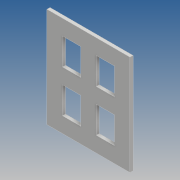
# Autodesk Inventor part: bandeja componentes
Saved by Autodesk Inventor 2017 (Build 210142000, 142)
## iProperties
Part Number: bandeja componentes
Material: Genérico
Document SubType Name: Modeling
Designer: FABLAB
Density: 1 g/cm^3
Appearance: Valor por defecto
Description: Aluminio compuesto routeado CNC
Author: FABLAB
Autodesk Inventor part; units mm, degrees
ref_plane "YZ Plane" through (0, 0, 0) normal (1, 0, 0) x (0, 1, 0)
ref_plane "XZ Plane" through (0, 0, 0) normal (0, 1, 0) x (-1, 0, 0)
ref_plane "XY Plane" through (0, 0, 0) normal (0, 0, 1) x (1, 0, 0)
sketch "Boceto1" plane through (0, 0, 0) normal (0, 1, 0) x (-1, 0, 0)
  line L0 (54, 65) -> (-54, 65)
  line L1 (-54, 65) -> (-54, -65)
  line L2 (-54, -65) -> (54, -65)
  line L3 (54, -65) -> (54, 65)
  line L4 (34, 45) -> (10, 45)
  line L5 (10, 45) -> (10, 10)
  line L6 (10, 10) -> (34, 10)
  line L7 (34, 10) -> (34, 45)
  line L8 (10, -10) -> (34, -10)
  line L9 (34, -10) -> (34, -45)
  line L10 (34, -45) -> (10, -45)
  line L11 (10, -45) -> (10, -10)
  line L12 (-10, -45) -> (-34, -45)
  line L13 (-34, -45) -> (-34, -10)
  line L14 (-34, -10) -> (-10, -10)
  line L15 (-10, -10) -> (-10, -45)
  line L16 (-34, 10) -> (-10, 10)
  line L17 (-10, 10) -> (-10, 45)
  line L18 (-10, 45) -> (-34, 45)
  line L19 (-34, 45) -> (-34, 10)
  line L20 (141.1986, 0) -> (-141.1986, 0) construction
  line L21 (0, -44.0939) -> (0, 44.0939) construction
  point P0 (0, 0)
  point P1 (54, 0)
  point P2 (0, -65)
  point P3 (0, 0)
  dimension "d0" = 108
  dimension "d1" = 130
  dimension "d2" = 20
  dimension "d3" = 20
  dimension "d4" = 20
  dimension "d5" = 20
  constraints: 44 end point, 10 parallel, 8 point on line, 6 horizontal, 5 perpendicular, 4 midpoint, 2 collinear, 1 coincident, 1 horizontal alignment, 1 vertical, 1 vertical alignment, 3 other
  measures "d0" distance of L1.end L2.end
  measures "d1" distance of L2.end L0.start
  measures "d2" diameter of L8 L20
  measures "d3" distance between parallel lines of L11 L15
  measures "d4" distance between parallel lines of L2 L10
  measures "d5" distance between parallel lines of L3 L9
extrude "Extrusión1" add sketch "Boceto1" along normal blind 4
equation "\"d3\" = d2"
equation "\"d4\" = d3"
equation "\"d5\" = d2"
